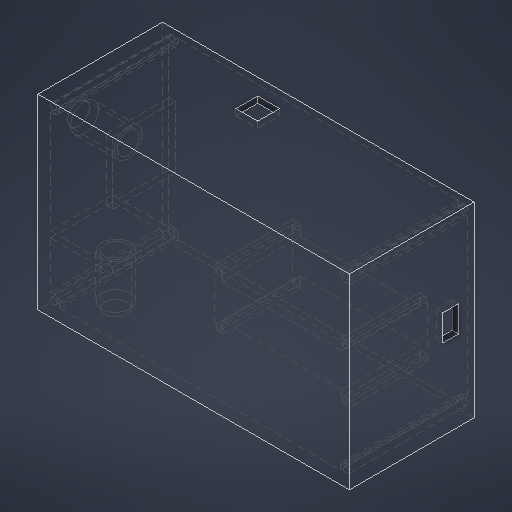
# Autodesk Inventor part: Part2
Saved by Autodesk Inventor 2026.2 (Build 302298000, 298)
## iProperties
Created: 2026-04-03
Part Number: Part2
Material: Generic
Document SubType Name: Modeling
Designer: Octa
Density: 1 g/cm^3
Appearance: Default
Author: Octa
Autodesk Inventor part; units mm, degrees
ref_plane "YZ Plane" through (0, 0, 0) normal (1, 0, 0) x (0, 1, 0)
ref_plane "XZ Plane" through (0, 0, 0) normal (0, 1, 0) x (-1, 0, 0)
ref_plane "XY Plane" through (0, 0, 0) normal (0, 0, 1) x (1, 0, 0)
sketch "Sketch1" plane through (0, 0, 0) normal (0, 0, 1) x (1, 0, 0)
  line L0 (-12.7529, 51.3281) -> (87.2471, 51.3281)
  line L1 (87.2471, 51.3281) -> (87.2471, -8.6719)
  line L2 (87.2471, -8.6719) -> (-12.7529, -8.6719)
  line L3 (-12.7529, -8.6719) -> (-12.7529, 51.3281)
  point P0 (0, 0)
  dimension "d0" = 100
  dimension "d1" = 60
  constraints: 8 end point, 2 parallel, 1 horizontal, 1 perpendicular
  measures "d0" distance of L1.end L2.end
  measures "d1" distance of L2.end L0.start
extrude "Extrusion1" add sketch "Sketch1" along normal blind 40
shell "Shell1" thickness 2 removed faces 1 at (20.5805, 31.3281, 0)
sketch "Sketch2" plane through (85.2471, -6.6719, 38) normal (0, 0, -1) x (-1, 0, 0)
  line L0 (0, 0) -> (0, 56) projected
  line L1 (43.2, 19) -> (43.2, 37)
  line L2 (0, 37) -> (0, 19)
  line L3 (43.2, 19) -> (40.7, 19)
  line L4 (40.7, 19) -> (40.7, 22.5)
  line L5 (0, 16.6053) -> (0, 19)
  line L6 (0, 19) -> (2.5, 19)
  line L7 (2.5, 19) -> (2.5, 22.5)
  line L8 (2.5, 22.5) -> (40.7, 22.5)
  line L9 (0, 19) -> (2.5, 19)
  line L10 (40.7, 19) -> (43.2, 19)
  line L11 (43.2, 37) -> (40.7, 37)
  line L12 (40.7, 37) -> (40.7, 33.5)
  line L13 (40.7, 33.5) -> (2.5, 33.5)
  line L14 (2.5, 33.5) -> (2.5, 37)
  line L15 (43.2, 37) -> (40.7, 37)
  line L16 (2.5, 37) -> (0, 37)
  line L17 (96, 0) -> (0, 0) projected
  circle A0 centre (41.92, 20.3797) radius 0.9
  circle A1 centre (41.95, 35.62) radius 0.9
  circle A2 centre (1.28, 20.38) radius 0.9
  circle A3 centre (1.25, 35.62) radius 0.9
  line L18 (0, 56) -> (96, 56) projected
  point P0 (85.2471, 6.6719)
  point P1 (1.25, 19)
  point P2 (41.95, 19)
  point P3 (0, 37)
  point P4 (1.25, 37)
  point P5 (1.25, 19)
  dimension "d5" = 43.2
  dimension "d6" = 18
  dimension "d7" = 2.5
  dimension "d8" = 3.5
  dimension "d9" = 2.5
  dimension "d10" = 3.5
  dimension "d12" = 3.5
  dimension "d13" = 1.8
  dimension "d14" = 1.38
  dimension "d15" = 1.28
  dimension "d16" = 1.8
  dimension "d17" = 1.8
  dimension "d18" = 1.8
  dimension "d19" = 1.38
  dimension "d20" = 1.28
  dimension "d29" = 1.38
  dimension "d30" = 1.25
  dimension "d31" = 3.5
  dimension "d32" = 19
  dimension "d33" = 1.38
  constraints: 32 end point, 10 perpendicular, 5 parallel, 4 centre point, 4 midpoint, 2 horizontal, 2 point on line, 1 collinear
  measures "d5" distance of L2.start L1.end
  measures "d6" distance of L1.end L1.start
  measures "d7" distance of L1.start L3.end
  measures "d8" distance of L3.end L4.end
  measures "d9" distance of L2.end L6.end
  measures "d10" distance of L11.end L12.end
  measures "d12" distance of L6.end L7.end
  measures "d13" diameter of A0
  measures "d14" distance of A0.centre point (41.95, 19)
  measures "d15" distance from line of A0.centre L1
  measures "d16" diameter of A1
  measures "d17" diameter of A2
  measures "d18" diameter of A3
  measures "d19" distance from line of L11 A1.centre
  measures "d20" distance from line of L2 A2.centre
  measures "d29" distance of point (1.25, 37) A3.centre
  measures "d30" distance from line of L14 A3.centre
  measures "d31" distance of L13.end L14.end
  measures "d32" distance between parallel lines of L18 L16
  measures "d33" vertical distance of point (1.25, 19) A2.centre
extrude "Extrusion2" add sketch "Sketch2" along normal blind 25
sketch "Sketch5" plane through (85.2471, -6.6719, 38) normal (0, 0, -1) x (-1, 0, 0)
  line L0 (0, 56) -> (96, 56) projected
  line L1 (77.9752, 56) -> (75.9752, 56)
  line L2 (75.9752, 56) -> (75.9752, 36)
  line L3 (75.9752, 36) -> (77.9752, 36)
  line L4 (77.9752, 36) -> (77.9752, 56)
  point P0 (85.2471, 6.6719)
  point P1 (75.9752, 56)
  dimension "d40" = 20
  dimension "d41" = 2
  constraints: 8 end point, 2 parallel, 1 horizontal, 1 perpendicular, 1 point on line
  measures "d40" distance of L3.end L1.start
  measures "d41" distance of L2.end L3.end
extrude "Extrusion5" add sketch "Sketch5" along normal blind 20
sketch "Sketch6" plane through (-12.7529, -8.6719, 0) normal (-1, 0, 0) x (0, 0, 1)
  circle A0 centre (27, 48) radius 3.5
  line L0 (18, 58) -> (18, 31.1645)
  line L1 (13, 23.2797) -> (38, 23.2797) projected
  line L2 (0, 58) -> (38, 58) projected
  point P0 (0, 8.6719)
  point P1 (18, 44.5822)
  dimension "d44" = 7
  dimension "d45" = 9
  dimension "d46" = 10
  constraints: 2 end point, 1 centre point, 1 midpoint, 1 perpendicular
  measures "d44" diameter of A0
  measures "d45" horizontal distance of A0.centre point (18, 44.582)
  measures "d46" distance from line of L2 A0.centre
extrude "Extrusion6" cut sketch "Sketch6" against normal blind 4
sketch "Sketch7" plane through (-10.7529, -6.6719, 0) normal (1, 0, 0) x (0, 0, -1)
  circle A0 centre (-27, 46) radius 4.5
  line L0 (-40, -2) -> (-40, 58) projected
  circle A1 centre (-27, 46) radius 3.5
  line L1 (0, 56) -> (-38, 56) projected
  point P0 (0, 6.6719)
  dimension "d49" = 9
  dimension "d50" = 13
  dimension "d51" = 7
  dimension "d52" = 10
  constraints: 2 centre point, 1 coincident
  measures "d49" diameter of A0
  measures "d50" distance from line of A0.centre L0
  measures "d51" diameter of A1
  measures "d52" distance from line of A0.centre L1
extrude "Extrusion7" add sketch "Sketch7" along normal blind 14
sketch "Sketch8" plane through (85.2471, -6.6719, 38) normal (0, 0, -1) x (-1, 0, 0)
  line L0 (96, 56) -> (96, 0) projected
  line L1 (96, 20.025) -> (76, 20.025)
  line L2 (76, 20.025) -> (76, 18.025)
  line L3 (76, 18.025) -> (96, 18.025)
  line L4 (96, 18.025) -> (96, 20.025)
  line L5 (96, 0) -> (0, 0) projected
  point P0 (85.2471, 6.6719)
  dimension "d55" = 20
  dimension "d56" = 2
  dimension "d57" = 18.025
  constraints: 8 end point, 2 parallel, 1 horizontal, 1 perpendicular, 1 point on line
  measures "d55" distance of L3.end L2.end
  measures "d56" distance of L2.end L1.end
  measures "d57" distance between parallel lines of L5 L3
extrude "Extrusion8" add sketch "Sketch8" along normal blind 20
sketch "Sketch9" plane through (-12.7529, -8.6719, 0) normal (0, -1, 0) x (1, 0, 0)
  circle A0 centre (12, 27) radius 3.5
  line L0 (0, 40) -> (100, 40) projected
  line L1 (2, 0) -> (2, 38) projected
  point P0 (12.7529, 0)
  dimension "d60" = 7
  dimension "d61" = 13
  dimension "d62" = 10
  constraints: 1 centre point
  measures "d60" diameter of A0
  measures "d61" distance from line of L0 A0.centre
  measures "d62" distance from line of A0.centre L1
extrude "Extrusion9" cut sketch "Sketch9" against normal blind 4
sketch "Sketch10" plane through (-10.7529, -6.6719, 0) normal (0, 1, 0) x (1, 0, 0)
  circle A0 centre (10, -27) radius 3.5
  line L0 (98, -40) -> (-2, -40) projected
  line L1 (-2, 0) -> (-2, -40) projected
  circle A1 centre (10, -27) radius 4.5
  point P0 (10.7529, 0)
  dimension "d65" = 7
  dimension "d66" = 13
  dimension "d67" = 12
  dimension "d68" = 9
  constraints: 2 centre point, 1 coincident
  measures "d65" diameter of A0
  measures "d66" distance from line of L0 A0.centre
  measures "d67" distance from line of L1 A0.centre
  measures "d68" diameter of A1
extrude "Extrusion10" add sketch "Sketch10" along normal blind 14
sketch "Sketch11" plane through (87.2471, -8.6719, 0) normal (1, 0, 0) x (0, 0, -1)
  line L0 (-5, 25.8) -> (-10, 25.8)
  line L1 (-10, 25.8) -> (-10, 34.2)
  line L2 (-10, 34.2) -> (-5, 34.2)
  line L3 (-5, 34.2) -> (-5, 25.8)
  line L4 (-40, 0) -> (-40, 60) projected
  line L5 (0, 0) -> (-40, 0) projected
  point P0 (0, 8.6719)
  dimension "d71" = 5
  dimension "d72" = 8.4
  dimension "d73" = 30
  dimension "d74" = 25.8
  constraints: 8 end point, 2 parallel, 1 horizontal, 1 perpendicular
  measures "d71" distance of L1.end L2.end
  measures "d72" distance of L0.end L1.end
  measures "d73" distance between parallel lines of L4 L1
  measures "d74" distance between parallel lines of L0 L5
extrude "Extrusion11" cut sketch "Sketch11" against normal blind 2
sketch "Sketch12" plane through (85.2471, -6.6719, 38) normal (0, 0, -1) x (-1, 0, 0)
  line L0 (96, 0) -> (0, 0) projected
  line L1 (96, 0) -> (93, 0)
  line L2 (93, 0) -> (93, 1)
  line L3 (95, 3) -> (96, 3)
  line L4 (96, 3) -> (96, 0)
  line L5 (96, 56.0056) -> (93, 56.0056)
  line L6 (93, 56.0056) -> (93, 55.0056)
  line L7 (95, 53.0056) -> (96, 53.0056)
  line L8 (96, 53.0056) -> (96, 56.0056)
  line L9 (0, 56.0056) -> (3, 56.0056)
  line L10 (3, 56.0056) -> (3, 55.0056)
  line L11 (1, 53.0056) -> (0, 53.0056)
  line L12 (0, 53.0056) -> (0, 56.0056)
  line L13 (0, 0) -> (3, 0)
  line L14 (3, 0) -> (3, 1)
  line L15 (1, 3) -> (0, 3)
  line L16 (0, 3) -> (0, 0)
  circle A0 centre (95, 55.0056) radius 1
  arc A1 (93, 55.0056) -> (95, 53.0056) centre (95, 55.0056) ccw
  arc A2 (95, 3) -> (93, 1) centre (95, 1) ccw
  arc A3 (1, 53.0056) -> (3, 55.0056) centre (1, 55.0056) ccw
  arc A4 (3, 1) -> (1, 3) centre (1, 1) ccw
  circle A5 centre (95, 1) radius 1
  circle A6 centre (1, 1) radius 1
  circle A7 centre (1, 55.0056) radius 1
  point P0 (85.2471, 6.6719)
  point P1 (93, 3)
  point P2 (93, 53.0056)
  point P3 (3, 53.0056)
  point P4 (3, 3)
  point P5 (0, 1)
  point P6 (1, 0)
  point P7 (3, 0)
  point P8 (1, 56.0056)
  point P9 (0, 55.0056)
  point P10 (95, 56.0056)
  point P11 (96, 55.0056)
  point P12 (96, 1)
  point P13 (95, 0)
  dimension "d77" = 3
  dimension "d78" = 3
  dimension "d79" = 3
  dimension "d80" = 3
  dimension "d81" = 3
  dimension "d82" = 3
  dimension "d83" = 3
  dimension "d84" = 2
  dimension "d85" = 0
  dimension "d86" = 1
  dimension "d87" = 2
  dimension "d88" = 2
  dimension "d89" = 2
  dimension "d90" = 2
  constraints: 32 end point, 9 point on line, 8 centre point, 8 parallel, 8 point on circle, 8 tangent, 4 horizontal, 4 perpendicular, 3 coincident, 3 equal radius
  measures "d77" distance of point (93, 3) L3.end
  measures "d78" distance of L1.end point (93, 3)
  measures "d79" distance of L7.end point (93, 53.006)
  measures "d80" distance of point (93, 53.006) L5.end
  measures "d81" distance of point (3, 53.006) L11.end
  measures "d82" distance of L9.end point (3, 53.006)
  measures "d83" distance of L15.end point (3, 3)
  measures "d84" diameter of A0
  measures "d85" distance edge to line of A0 L8
  measures "d86" distance from line of L5 A0.centre
  measures "d87" radius of A1
  measures "d88" diameter of A5
  measures "d89" diameter of A6
  measures "d90" diameter of A7
extrude "Extrusion12" add sketch "Sketch12" along normal blind 38 contours L0 A6 L16 L15 A4 L14 | L2 A2 L3 L4 A5 L0 | A5 L4 L0 | L0 L16 A6 | L8 A0 L5 | A0 L8 L7 A1 L6 L5 | L9 A7 L12 | L9 L10 A3 L11 L12 A7
sketch "Sketch13" plane through (-12.7529, 51.3281, 0) normal (0, 1, 0) x (1, 0, 0)
  line L0 (35.7867, -12.2294) -> (42.7867, -12.2294)
  line L1 (42.7867, -12.2294) -> (42.7867, -5.2294)
  line L2 (42.7867, -5.2294) -> (35.7867, -5.2294)
  line L3 (35.7867, -5.2294) -> (35.7867, -12.2294)
  point P0 (12.7529, 0)
  dimension "d93" = 7
  dimension "d94" = 7
  constraints: 8 end point, 2 parallel, 1 horizontal, 1 perpendicular
  measures "d93" distance of L2.end L1.end
  measures "d94" distance of L1.end L0.end
extrude "Extrusion13" cut sketch "Sketch13" against normal blind 10
body "Solid1"
